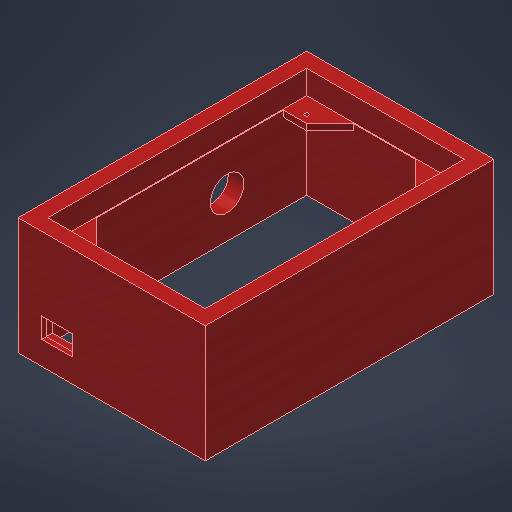
# Autodesk Inventor part: Enclose Top
Saved by Autodesk Inventor 2025.2 (Build 292293000, 293)
## iProperties
Created: 2025-03-24
Part Number: Enclose Top
Material: PC/ABS Plastic
Document SubType Name: Modeling
Designer: EJErickson
Density: 0.357273 g/cm^3
Appearance: Light Red
Author: EJErickson
Autodesk Inventor part; units mm, degrees
ref_plane "YZ Plane" through (0, 0, 0) normal (1, 0, 0) x (0, 1, 0)
ref_plane "XZ Plane" through (0, 0, 0) normal (0, 1, 0) x (-1, 0, 0)
sketch "Sketch1" plane through (0, 0, 0) normal (0, 1, 0) x (-1, 0, 0)
  line L0 (-50, 82.5) -> (50, 82.5)
  line L1 (50, 82.5) -> (50, -82.5)
  line L2 (50, -82.5) -> (-50, -82.5)
  line L3 (-50, -82.5) -> (-50, 82.5)
  line L4 (-50, 82.5) -> (50, -82.5) construction
  line L5 (50, 82.5) -> (-50, -82.5) construction
  line L6 (-60, 92.5) -> (60, 92.5)
  line L7 (60, 92.5) -> (60, -92.5)
  line L8 (60, -92.5) -> (-60, -92.5)
  line L9 (-60, -92.5) -> (-60, 92.5)
  line L10 (-60, 92.5) -> (60, -92.5) construction
  line L11 (60, 92.5) -> (-60, -92.5) construction
  point P0 (0, 0)
  dimension "d0" = 100
  dimension "d1" = 165
  dimension "d2" = 120
  dimension "d3" = 185
  constraints: 24 end point, 4 midpoint, 4 parallel, 2 horizontal, 2 perpendicular
  measures "d0" distance of L1.end L2.end
  measures "d1" distance of L0.end L1.end
  measures "d2" distance of L7.end L8.end
  measures "d3" distance of L6.end L7.end
extrude "Extrusion1" add sketch "Sketch1" along normal blind 75
ref_plane "Work Plane2" through (0, 59.8, 0) normal (0, 1, 0) x (1, 0, 0)
sketch "Sketch3" plane through (0, 59.8, 0) normal (0, 1, 0) x (1, 0, 0)
  line L0 (50, 82.5) -> (50, -82.5) projected
  line L1 (50, 82.5) -> (20, 82.5)
  line L2 (-50, 82.5) -> (50, 82.5) projected
  line L3 (50, 82.5) -> (50, 52.5)
  line L4 (50, 52.5) -> (20, 82.5)
  line L5 (50, -82.5) -> (50, -52.5)
  line L6 (50, -52.5) -> (20, -82.5)
  line L7 (50, -82.5) -> (-50, -82.5) projected
  line L8 (20, -82.5) -> (50, -82.5)
  line L9 (0, 82.5) -> (0, -82.5)
  line L10 (-50, 82.5) -> (-50, -82.5)
  line L11 (-50, 82.5) -> (-20, 82.5)
  line L12 (-50, 52.5) -> (-20, 82.5)
  line L13 (-50, -52.5) -> (-20, -82.5)
  line L14 (-50, -82.5) -> (50, -82.5)
  point P0 (0, 0)
  point P1 (-20, 82.5)
  dimension "d9" = 30
  dimension "d10" = 30
  dimension "d20" = 30
  dimension "d50" = 30
  constraints: 24 end point, 6 symmetric about line, 5 point on line, 2 midpoint, 1 collinear
  measures "d9" distance of L0.start L1.end
  measures "d10" distance of L0.start L3.end
  measures "d20" distance of L0.end L5.end
  measures "d50" distance of L0.end L6.end
extrude "Extrusion3" add sketch "Sketch3" against normal blind 4 contours L0 L4 L1 | L0 L7 L6 | L12 L10 L2 | L7 L10 L13
sketch "Sketch5" plane through (0, 59.8, 0) normal (0, 1, 0) x (1, 0, 0)
  circle A0 centre (40, 72.5) radius 1.3
  line L0 (50, 82.5) -> (50, -82.5) projected
  line L1 (50, 0) -> (-50, 0)
  line L2 (-50, -82.5) -> (-50, 82.5) projected
  line L3 (50, -82.5) -> (-50, -82.5) projected
  line L4 (0, -82.5) -> (0, 82.5)
  line L5 (-50, 82.5) -> (50, 82.5) projected
  line L6 (50, -82.5) -> (20, -82.5) projected
  line L7 (50, -82.5) -> (40, -82.5)
  line L8 (40, -82.5) -> (40, -72.5)
  line L9 (40, -72.5) -> (50, -72.5)
  line L10 (50, -72.5) -> (50, -82.5)
  circle A1 centre (40, -72.5) radius 1.3
  line L11 (-50, 52.5) -> (-50, 82.5) projected
  line L12 (-50, 82.5) -> (-40, 82.5)
  line L13 (-40, 82.5) -> (-40, 72.5)
  line L14 (-40, 72.5) -> (-50, 72.5)
  line L15 (-50, 72.5) -> (-50, 82.5)
  circle A2 centre (-40, 72.5) radius 1.3
  line L16 (-50, -82.5) -> (-40, -82.5)
  line L17 (-40, -82.5) -> (-40, -72.5)
  line L18 (-40, -72.5) -> (-50, -72.5)
  line L19 (-50, -72.5) -> (-50, -82.5)
  circle A3 centre (-40, -72.5) radius 1.3
  dimension "d17" = 2.6
  dimension "d21" = 10
  dimension "d22" = 10
  dimension "d23" = 2.6
  dimension "d24" = 10
  dimension "d25" = 10
  dimension "d26" = 2.6
  dimension "d27" = 10
  dimension "d28" = 10
  dimension "d29" = 2.6
  dimension "d48" = 10
  dimension "d49" = 10
  constraints: 28 end point, 6 parallel, 4 centre point, 4 midpoint, 3 coincident, 3 horizontal, 3 perpendicular
  measures "d17" diameter of A0
  measures "d21" distance of L8.end L9.end
  measures "d22" distance of L7.end L8.end
  measures "d23" diameter of A1
  measures "d24" distance of L13.end L14.end
  measures "d25" distance of L12.end L13.end
  measures "d26" diameter of A2
  measures "d27" distance of L18.end L17.end
  measures "d28" distance of L17.end L16.end
  measures "d29" diameter of A3
  measures "d48" distance from line of L0 A0.centre
  measures "d49" distance from line of L5 A0.centre
extrude "Extrusion5" cut sketch "Sketch5" against normal blind 4 contours A0 | A1 L8 L9 | L9 L8 A1 | A2 L14 L13 | L13 L14 A2 | A3 L17 L18 | L18 L17 A3
sketch "Sketch10" plane through (0, 0, 0) normal (0, -1, 0) x (1, 0, 0)
  line L0 (55, -87.5) -> (-55, -87.5)
  line L1 (-55, -87.5) -> (-55, 87.5)
  line L2 (-55, 87.5) -> (55, 87.5)
  line L3 (55, 87.5) -> (55, -87.5)
  line L4 (55, -87.5) -> (-55, 87.5) construction
  line L5 (-55, -87.5) -> (55, 87.5) construction
  point P0 (0, 0)
  dimension "d38" = 110
  dimension "d39" = 175
  constraints: 12 end point, 2 midpoint, 2 parallel, 1 horizontal, 1 perpendicular
  measures "d38" distance of L1.end L2.end
  measures "d39" distance of L0.end L1.end
extrude "Extrusion8" cut sketch "Sketch10" against normal blind 5
sketch "Sketch11" plane through (0, 0, 0) normal (0, -1, 0) x (1, 0, 0)
  line L0 (-55, -87.5) -> (-55, 87.5) projected
  line L1 (-60, -92.5) -> (-60, 92.5) projected
  circle A0 centre (-57.5, -90) radius 0.75
  line L2 (-60, -92.5) -> (-60, 92.5) projected
  circle A1 centre (-57.5, 90) radius 0.75
  line L3 (-60, 92.5) -> (60, 92.5) projected
  line L4 (55, 87.5) -> (55, -87.5) projected
  circle A2 centre (57.5, 90) radius 0.75
  line L5 (60, -92.5) -> (-60, -92.5) projected
  circle A3 centre (57.5, -90) radius 0.75
  point P0 (0, 0)
  dimension "d42" = 1.5
  dimension "d43" = 1.5
  dimension "d44" = 1.5
  dimension "d45" = 1.5
  constraints: 4 centre point
  measures "d42" diameter of A0
  measures "d43" diameter of A1
  measures "d44" diameter of A2
  measures "d45" diameter of A3
extrude "Extrusion9" cut sketch "Sketch11" against normal blind 5
sketch "Sketch12" plane through (0, 75, 0) normal (0, 1, 0) x (1, 0, 0)
  line L0 (-50.5, 83) -> (50.5, 83)
  line L1 (50.5, 83) -> (50.5, -83)
  line L2 (50.5, -83) -> (-50.5, -83)
  line L3 (-50.5, -83) -> (-50.5, 83)
  line L4 (-50.5, 83) -> (50.5, -83) construction
  line L5 (50.5, 83) -> (-50.5, -83) construction
  point P0 (0, 0)
  dimension "d51" = 101
  dimension "d52" = 166
  constraints: 12 end point, 2 midpoint, 2 parallel, 1 horizontal, 1 perpendicular
  measures "d51" distance of L1.end L2.end
  measures "d52" distance of L0.end L1.end
extrude "Extrusion10" cut sketch "Sketch12" against normal blind 15.2
sketch "Sketch15" plane through (0, 59.8, 0) normal (0, 1, 0) x (1, 0, 0)
  line L0 (-20, 82.5) -> (-50, 52.5) projected
  line L1 (-50, 52.5) -> (-50, 67.5)
  line L2 (-50, 67.5) -> (-35, 67.5)
  line L3 (-35, 67.5) -> (-35, 52.5)
  line L4 (-35, 52.5) -> (-50, 52.5)
  line L5 (-50, 52.5) -> (-50, 67.5)
  point P0 (0, 0)
  dimension "d56" = 15
  dimension "d57" = 15
  dimension "d58" = 15
  constraints: 10 end point, 2 parallel, 1 horizontal, 1 perpendicular, 1 vertical
  measures "d56" distance of L0.end L1.end
  measures "d57" distance of L3.end L4.end
  measures "d58" distance of L2.end L3.end
extrude "Extrusion11" cut sketch "Sketch15" against normal blind 4
sketch "Sketch16" plane through (-60, 0, 92.5) normal (0, 0, 1) x (1, 0, 0)
  line L0 (0, 0) -> (0, 75) projected
  line L1 (0, 0) -> (0, 15)
  line L2 (0, 15) -> (15, 15)
  line L3 (15, 15) -> (34.6, 15)
  line L4 (34.6, 15) -> (34.6, 28)
  line L5 (34.6, 28) -> (15, 28)
  line L6 (15, 28) -> (15, 15)
  point P0 (60, 0)
  dimension "d61" = 15
  dimension "d62" = 15
  dimension "d63" = 19.6
  dimension "d64" = 13
  constraints: 12 end point, 2 parallel, 2 perpendicular, 1 horizontal, 1 point on line
  measures "d61" distance of L0.start L1.end
  measures "d62" distance of L1.end L2.end
  measures "d63" distance of L5.end L4.end
  measures "d64" distance of L4.end L3.end
extrude "Extrusion12" cut sketch "Sketch16" against normal blind 10
sketch "Sketch18" plane through (20, 59.8, 82.5) normal (0, 0, -1) x (-1, 0, 0)
  line L0 (45.4, -44.8) -> (45.4, -31.8) projected
  line L1 (45.4, -31.8) -> (45.4, -28.8)
  line L2 (45.4, -28.8) -> (42.4, -28.8)
  line L3 (65, -31.8) -> (65, -44.8) projected
  line L4 (65, -44.8) -> (68, -44.8)
  line L5 (68, -44.8) -> (68, -47.8)
  line L6 (42.4, -28.8) -> (68, -28.8)
  line L7 (68, -28.8) -> (68, -47.8)
  line L8 (68, -47.8) -> (42.4, -47.8)
  line L9 (42.4, -47.8) -> (42.4, -28.8)
  point P0 (20, -59.8)
  dimension "d67" = 3
  dimension "d68" = 3
  dimension "d69" = 3
  dimension "d70" = 3
  constraints: 16 end point, 3 perpendicular, 2 horizontal, 2 parallel, 1 vertical
  measures "d67" distance of L0.end L1.end
  measures "d68" distance of L1.end L2.end
  measures "d69" distance of L3.end L4.end
  measures "d70" distance of L4.end L5.end
extrude "Extrusion13" cut sketch "Sketch18" against normal blind 7
sketch "Sketch19" plane through (-50, 55.8, 82.5) normal (1, 0, 0) x (0, 0, -1)
  line L0 (0, -50.8) -> (165, -50.8) projected
  circle A0 centre (114, -24.3) radius 10.75
  point P0 (82.5, -55.8)
  point P1 (114, -50.8)
  dimension "d73" = 51
  dimension "d74" = 26.5
  dimension "d75" = 21.5
  constraints: 1 centre point, 1 coincident, 1 point on line
  measures "d73" distance of L0.end point (114, -50.8)
  measures "d74" distance of point (114, -24.3) point (114, -50.8)
  measures "d75" diameter of A0
extrude "Extrusion14" cut sketch "Sketch19" against normal blind 10
body "Solid1"
